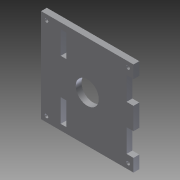
# Autodesk Inventor part: wheel top
Saved by Autodesk Inventor 2011 (Build 150239000, 239)
## iProperties
Created: 2011-02-20
Part Number: wheel top
Document SubType Name: Modeling
Designer: adowning
Density: 1 g/cm^3
Author: adowning
Autodesk Inventor part; units mm, degrees
ref_plane "YZ Plane" through (0, 0, 0) normal (1, 0, 0) x (0, 1, 0)
ref_plane "XZ Plane" through (0, 0, 0) normal (0, 1, 0) x (-1, 0, 0)
ref_plane "XY Plane" through (0, 0, 0) normal (0, 0, 1) x (1, 0, 0)
sketch "Sketch1" plane through (0, 0, 0) normal (0, 0, 1) x (1, 0, 0)
  line L0 (-26.62, 18.8707) -> (74.98, 18.8707)
  line L1 (74.98, 18.8707) -> (74.98, 12.5207)
  line L2 (74.98, -83.9993) -> (-26.62, -83.9993)
  line L3 (-26.62, -83.9993) -> (-26.62, 18.8707)
  line L4 (-26.62, 18.8707) -> (24.18, 18.8707)
  line L5 (24.18, 18.8707) -> (24.18, -33.1993)
  line L6 (24.18, -33.1993) -> (1.32, -33.1993)
  line L7 (24.18, -33.1993) -> (67.36, -33.1993)
  line L8 (1.32, -33.1993) -> (1.32, 12.5207)
  line L9 (1.32, 12.5207) -> (67.36, 12.5207)
  line L10 (67.36, 12.5207) -> (67.36, -33.1993)
  circle A0 centre (24.18, -33.1993) radius 12.7
  line L11 (74.98, 18.8707) -> (82.6, 18.8707)
  line L12 (82.6, 18.8707) -> (82.6, -83.9993)
  line L13 (82.6, -83.9993) -> (74.98, -83.9993)
  line L14 (1.32, -33.1993) -> (1.32, -77.6493)
  line L15 (1.32, 12.5207) -> (-5.03, 12.5207)
  line L16 (-5.03, 12.5207) -> (-5.03, -12.8793)
  line L17 (-5.03, -12.8793) -> (1.32, -12.8793)
  line L18 (1.32, -77.6493) -> (-5.03, -77.6493)
  line L19 (-5.03, -77.6493) -> (-5.03, -52.2493)
  line L20 (-5.03, -52.2493) -> (1.32, -52.2493)
  line L21 (1.32, -77.6493) -> (1.32, -45.2643)
  line L22 (1.32, -45.2643) -> (-5.03, -45.2643)
  line L23 (-5.03, -45.2643) -> (-5.03, -19.8643)
  line L24 (-5.03, -19.8643) -> (1.32, -19.8643)
  line L25 (67.36, -33.1993) -> (67.36, -77.6493)
  line L26 (67.36, -77.6493) -> (73.71, -77.6493)
  line L27 (73.71, -77.6493) -> (73.71, -52.2493)
  line L28 (73.71, -52.2493) -> (67.36, -52.2493)
  line L29 (67.36, -52.2493) -> (67.36, -45.2643)
  line L30 (67.36, -45.2643) -> (73.71, -45.2643)
  line L31 (73.71, -45.2643) -> (73.71, -19.8643)
  line L32 (73.71, -19.8643) -> (67.36, -19.8643)
  line L33 (67.36, 12.5207) -> (73.71, 12.5207)
  line L34 (73.71, 12.5207) -> (73.71, -12.8793)
  line L35 (73.71, -12.8793) -> (67.36, -12.8793)
  point P0 (0, 0)
  dimension "d0" = 101.6
  dimension "d1" = 102.87
  dimension "d2" = 50.8
  dimension "d3" = 52.07
  dimension "d4" = 22.86
  dimension "d5" = 43.18
  dimension "d6" = 45.72
  dimension "d7" = 25.4
  dimension "d8" = 7.62
  dimension "d9" = 44.45
  dimension "d10" = 6.35
  dimension "d11" = 25.4
  dimension "d12" = 6.35
  dimension "d13" = 25.4
  dimension "d14" = 32.385
  dimension "d15" = 25.4
  dimension "d16" = 6.35
  dimension "d17" = 25.4
  dimension "d18" = 6.985
  dimension "d19" = 25.4
  constraints: 72 end point, 22 perpendicular, 10 point on line, 8 parallel, 1 centre point, 1 coincident, 1 collinear, 1 horizontal, 1 midpoint
  measures "d0" distance of L2.start L2.end
  measures "d1" distance of L0.end L2.start
  measures "d2" distance of L0.start L4.end
  measures "d3" distance of L4.end L5.end
  measures "d4" distance of L5.end L6.end
  measures "d5" distance of L5.end L7.end
  measures "d6" distance of L6.end L8.end
  measures "d7" diameter of A0
  measures "d8" distance of L0.end L11.end
  measures "d9" distance of L6.end L14.end
  measures "d10" distance of L8.end L15.end
  measures "d11" distance of L15.end L16.end
  measures "d12" distance of L14.end L18.end
  measures "d13" distance of L18.end L19.end
  measures "d14" distance of L14.end L21.end
  measures "d15" distance of L22.end L23.end
  measures "d16" distance of L25.end L26.end
  measures "d17" distance of L26.end L27.end
  measures "d18" distance of L28.end L29.end
  measures "d19" distance of L30.end L31.end
extrude "Extrusion1" add sketch "Sketch1" along normal blind 6.35 contours L0 L11 L12 L13 L2 L3 | L9 L10 L7 A0 L5 | L5 A0 L6 L8 L9
sketch "Sketch2" plane through (0, 0, 6.35) normal (0, 0, 1) x (1, 0, 0)
  arc A0 (11.48, -33.1993) -> (36.88, -33.1993) centre (24.18, -33.1993) ccw projected
  line L0 (36.88, -33.1993) -> (11.48, -33.1993) projected
  circle A1 centre (24.18, -33.1993) radius 12.7
  point P0 (0, 0)
  dimension "d22" = 25.4
  constraints: 1 centre point, 1 coincident
  measures "d22" diameter of A1
extrude "Extrusion2" cut sketch "Sketch2" against normal blind 6.35 contours A1 L0
sketch "Sketch3" plane through (0, 0, 6.35) normal (0, 0, 1) x (1, 0, 0)
  line L0 (-26.62, 18.8707) -> (82.6, 18.8707) projected
  line L1 (82.6, -83.9993) -> (-26.62, -83.9993) projected
  line L2 (-26.62, 18.8707) -> (-20.6637, 18.8707)
  line L3 (-20.6637, 18.8707) -> (-20.6637, 12.9144)
  line L4 (-26.62, -83.9993) -> (-20.6637, -83.9993)
  line L5 (-20.6637, -83.9993) -> (-20.6637, -78.043)
  line L6 (-26.62, 18.8707) -> (74.98, 18.8707)
  circle A0 centre (-20.6637, 12.9144) radius 1.9812
  circle A1 centre (-20.6637, -78.043) radius 1.9812
  point P0 (0, 0)
  dimension "d25" = 5.9563
  dimension "d26" = 5.9563
  dimension "d27" = 5.9563
  dimension "d28" = 5.9563
  dimension "d29" = 101.6
  dimension "d30" = 3.9624
  dimension "d31" = 3.9624
  constraints: 10 end point, 3 point on line, 2 centre point, 2 coincident, 2 perpendicular
  measures "d25" distance of L0.start L2.end
  measures "d26" distance of L2.end L3.end
  measures "d27" distance of L1.end L4.end
  measures "d28" distance of L4.end L5.end
  measures "d29" distance of L0.start L6.end
  measures "d30" diameter of A0
  measures "d31" diameter of A1
extrude "Extrusion3" cut sketch "Sketch3" against normal blind 6.35
sketch "Sketch4" plane through (0, 0, 6.35) normal (0, 0, 1) x (1, 0, 0)
  line L0 (67.36, 12.5207) -> (73.71, 12.5207) projected
  line L1 (73.71, 12.5207) -> (73.71, -12.8793) projected
  line L2 (67.36, -12.8793) -> (67.36, 12.5207) projected
  line L3 (1.32, 12.5207) -> (1.32, -12.8793) projected
  line L4 (-5.03, -12.8793) -> (-5.03, 12.5207) projected
  line L5 (-5.03, 12.5207) -> (1.32, 12.5207) projected
  line L6 (-5.03, 12.5207) -> (-5.03, -0.1793)
  line L7 (-5.03, -0.1793) -> (1.32, -0.1793)
  line L8 (67.36, 12.5207) -> (67.36, -0.1793)
  line L9 (67.36, -0.1793) -> (73.71, -0.1793)
  point P0 (0, 0)
  dimension "d34" = 12.7
  dimension "d35" = 12.7
  constraints: 8 end point, 4 midpoint
  measures "d34" distance of L4.end L6.end
  measures "d35" distance of L0.start L8.end
extrude "Extrusion4" add sketch "Sketch4" against normal blind 6.35
sketch "Sketch5" plane through (0, 0, 6.35) normal (0, 0, 1) x (1, 0, 0)
  circle A0 centre (-20.6637, 12.9144) radius 1.9812 projected
  line L0 (-26.62, 18.8707) -> (82.6, 18.8707) projected
  line L1 (82.6, -83.9993) -> (-26.62, -83.9993) projected
  line L2 (73.71, -52.2493) -> (73.71, -77.6493) projected
  line L3 (67.36, -77.6493) -> (67.36, -52.2493) projected
  line L4 (67.36, -0.1793) -> (73.71, -0.1793) projected
  line L5 (-5.03, -0.1793) -> (1.32, -0.1793) projected
  line L6 (-26.62, 18.8707) -> (74.98, 18.8707)
  line L7 (74.98, 18.8707) -> (74.98, 12.9144)
  line L8 (-26.62, -83.9993) -> (74.98, -83.9993)
  line L9 (-5.03, -0.1793) -> (-5.03, 12.5207)
  line L10 (-5.03, 12.5207) -> (1.32, 12.5207)
  line L11 (1.32, 12.5207) -> (1.32, -0.1793)
  line L12 (67.36, -77.6493) -> (67.36, -70.0293)
  line L13 (67.36, -70.0293) -> (73.71, -70.0293)
  line L14 (67.36, -0.1793) -> (67.36, 4.9007)
  line L15 (67.36, 4.9007) -> (73.71, 4.9007)
  line L16 (73.71, 4.9007) -> (73.71, -0.1793)
  point P0 (0, 0)
  dimension "d38" = 101.6
  dimension "d39" = 5.9563
  dimension "d40" = 5.9563
  dimension "d41" = 101.6
  dimension "d42" = 12.7
  dimension "d43" = 7.62
  dimension "d44" = 5.08
  constraints: 22 end point, 7 perpendicular, 4 point on line, 1 parallel
  measures "d38" distance of L0.start L6.end
  measures "d39" distance from line of L6 A0.centre
  measures "d40" distance of L6.end L7.end
  measures "d41" distance of L1.end L8.end
  measures "d42" distance of L5.start L9.end
  measures "d43" distance of L3.start L12.end
  measures "d44" distance of L4.start L14.end
extrude "Extrusion5" cut sketch "Sketch5" against normal blind 6.35 contours L14 L15 L16 L4 | L9 L10 L11 L5
sketch "Sketch6" plane through (0, 0, 6.35) normal (0, 0, 1) x (1, 0, 0)
  line L0 (73.71, -52.2493) -> (73.71, -77.6493) projected
  line L1 (73.71, -77.6493) -> (67.36, -77.6493) projected
  line L2 (67.36, -77.6493) -> (67.36, -52.2493) projected
  line L3 (67.36, -77.6493) -> (67.36, -70.0293)
  line L4 (67.36, -70.0293) -> (73.71, -70.0293)
  point P0 (0, 0)
  dimension "d47" = 7.62
  constraints: 4 end point, 2 point on line, 1 perpendicular
  measures "d47" distance of L1.end L3.end
extrude "Extrusion6" add sketch "Sketch6" against normal blind 6.35
sketch "Sketch7" plane through (0, 0, 6.35) normal (0, 0, 1) x (1, 0, 0)
  line L0 (-26.62, 18.8707) -> (82.6, 18.8707) projected
  line L1 (82.6, -83.9993) -> (-26.62, -83.9993) projected
  line L2 (-26.62, 18.8707) -> (74.98, 18.8707)
  line L3 (74.98, 18.8707) -> (74.98, 12.9144)
  line L4 (-26.62, -83.9993) -> (74.98, -83.9993)
  line L5 (74.98, -83.9993) -> (74.98, -78.043)
  line L6 (74.98, -78.043) -> (69.0237, -78.043)
  line L7 (74.98, 12.9144) -> (69.0237, 12.9144)
  circle A0 centre (69.0237, 12.9144) radius 1.9812
  circle A1 centre (69.0237, -78.043) radius 1.9812
  point P0 (0, 0)
  dimension "d50" = 101.6
  dimension "d51" = 5.9563
  dimension "d52" = 101.6
  dimension "d53" = 5.9563
  dimension "d54" = 5.9563
  dimension "d55" = 5.9563
  dimension "d56" = 3.9624
  dimension "d57" = 3.9624
  constraints: 12 end point, 2 centre point, 2 coincident, 2 parallel, 2 perpendicular, 2 point on line
  measures "d50" distance of L0.start L2.end
  measures "d51" distance of L2.end L3.end
  measures "d52" distance of L1.end L4.end
  measures "d53" distance of L4.end L5.end
  measures "d54" distance of L5.end L6.end
  measures "d55" distance of L3.end L7.end
  measures "d56" diameter of A0
  measures "d57" diameter of A1
extrude "Extrusion7" cut sketch "Sketch7" against normal blind 6.35
sketch "Sketch8" plane through (0, 0, 6.35) normal (0, 0, 1) x (1, 0, 0)
  line L0 (73.71, 4.9007) -> (73.71, -12.8793) projected
  line L1 (-26.62, 18.8707) -> (82.6, 18.8707) projected
  line L2 (82.6, -83.9993) -> (-26.62, -83.9993) projected
  line L3 (82.6, 18.8707) -> (82.6, -83.9993) projected
  line L4 (73.71, -52.2493) -> (73.71, -70.0293) projected
  line L5 (73.71, -19.8643) -> (73.71, -45.2643) projected
  line L6 (-26.62, 18.8707) -> (74.98, 18.8707)
  line L7 (74.98, 18.8707) -> (74.98, -83.9993)
  line L8 (73.71, -52.2493) -> (74.98, -52.2493)
  line L9 (73.71, -70.0293) -> (74.98, -70.0293)
  line L10 (73.71, -45.2643) -> (74.98, -45.2643)
  line L11 (73.71, -19.8643) -> (74.98, -19.8643)
  line L12 (73.71, 4.9007) -> (74.98, 4.9007)
  line L13 (73.71, -12.8793) -> (74.98, -12.8793)
  point P0 (0, 0)
  dimension "d60" = 101.6
  constraints: 16 end point, 8 point on line, 5 perpendicular, 2 parallel
  measures "d60" distance of L1.start L6.end
extrude "Extrusion8" cut sketch "Sketch8" against normal blind 6.35
sketch "Sketch9" plane through (0, 0, 6.35) normal (0, 0, 1) x (1, 0, 0)
  line L0 (74.98, -45.2643) -> (67.36, -45.2643) projected
  line L1 (67.36, -45.2643) -> (67.36, -19.8643) projected
  line L2 (67.36, -19.8643) -> (74.98, -19.8643) projected
  line L3 (-5.03, 12.5207) -> (1.32, 12.5207) projected
  line L4 (74.98, -19.8643) -> (74.98, -45.2643)
  point P0 (0, 0)
  constraints: 2 end point, 1 perpendicular
extrude "Extrusion9" add sketch "Sketch9" against normal blind 6.35
sketch "Sketch11" plane through (0, 0, 6.35) normal (0, 0, 1) x (1, 0, 0)
  line L0 (67.36, 4.9007) -> (74.98, 4.9007) projected
  line L1 (74.98, -83.9993) -> (74.98, -70.0293) projected
  line L2 (67.36, -70.0293) -> (67.36, -52.2493) projected
  line L3 (74.98, -52.2493) -> (74.98, -12.8793) projected
  line L4 (67.36, -12.8793) -> (67.36, 4.9007) projected
  line L5 (-5.03, 12.5207) -> (1.32, 12.5207) projected
  line L6 (67.36, 4.9007) -> (67.36, -20.4993)
  line L7 (67.36, -20.4993) -> (74.98, -20.4993)
  line L8 (74.98, 4.9007) -> (74.98, -20.4993)
  line L9 (74.98, 4.9007) -> (67.36, 4.9007)
  line L10 (67.36, -70.0293) -> (67.36, -44.6293)
  line L11 (67.36, -44.6293) -> (74.98, -44.6293)
  line L12 (74.98, -44.6293) -> (74.98, -70.0293)
  line L13 (67.36, -70.0293) -> (74.98, -70.0293)
  point P0 (0, 0)
  dimension "d67" = 25.4
  dimension "d68" = 25.4
  dimension "d69" = 7.62
  constraints: 16 end point, 4 perpendicular, 3 point on line, 2 collinear
  measures "d67" distance of L0.start L6.end
  measures "d68" distance of L2.start L10.end
  measures "d69" distance of L10.end L11.end
extrude "Extrusion10" cut sketch "Sketch11" against normal blind 6.35
sketch "Sketch12" plane through (0, 0, 6.35) normal (0, 0, 1) x (1, 0, 0)
  line L0 (1.32, -19.8643) -> (1.32, -45.2643) projected
  line L1 (1.32, -45.2643) -> (-5.03, -45.2643) projected
  line L2 (-5.03, -45.2643) -> (-5.03, -19.8643) projected
  line L3 (-5.03, -19.8643) -> (1.32, -19.8643) projected
  point P0 (0, 0)
extrude "Extrusion11" add sketch "Sketch12" against normal blind 6.35
body "Solid1"
